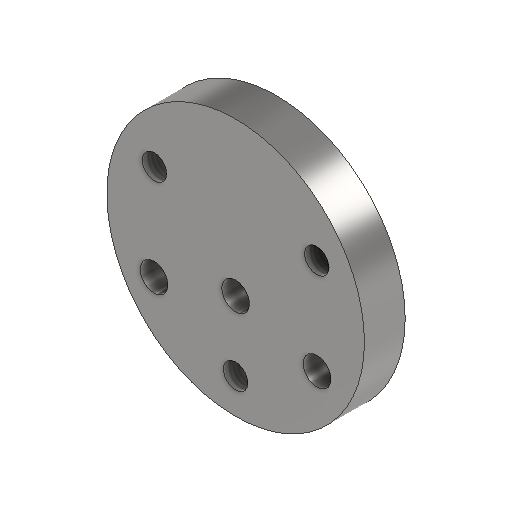
# Autodesk Inventor part: B_pipe_cylinder_5
Saved by Autodesk Inventor 2026.2 (Build 302298000, 298)
## iProperties
Created: 2026-02-02
Part Number: B_pipe_cylinder_5
Material: ステンレス鋼 440C
Document SubType Name: Modeling
Designer: zetsu
Density: 7.75 g/cm^3
Appearance: 半つや出し
Author: zetsu
Autodesk Inventor part; units mm, degrees
ref_plane "YZ Plane" through (0, 0, 0) normal (1, 0, 0) x (0, 1, 0)
ref_plane "XZ Plane" through (0, 0, 0) normal (0, 1, 0) x (-1, 0, 0)
ref_plane "XY Plane" through (0, 0, 0) normal (0, 0, 1) x (1, 0, 0)
sketch "スケッチ2" plane through (0, 0, 0) normal (0, 0, 1) x (1, 0, 0)
  circle A0 centre (0, 0) radius 15.8
  dimension "d0" = 31.6
  constraints: 1 centre point, 1 coincident
  measures "d0" diameter of A0
extrude "押し出し1" add sketch "スケッチ2" against normal blind 5
sketch "スケッチ3" plane through (0, 0, 0) normal (0, 0, 1) x (1, 0, 0)
  line L0 (0, 0) -> (0, 20.2537) construction
  circle A0 centre (0, -3) radius 1.7
  circle A1 centre (-10, -6) radius 1.7
  circle A2 centre (10, -6) radius 1.7
  dimension "d32" = 3.4
  dimension "d33" = 3
  dimension "d67" = 3.4
  dimension "d68" = 3.4
  dimension "d69" = 10
  dimension "d70" = 6
  constraints: 3 centre point, 2 end point, 1 symmetric about line, 1 vertical
  measures "d32" diameter of A0
  measures "d33" distance of A0.centre L0.start
  measures "d67" diameter of A1
  measures "d68" diameter of A2
  measures "d69" horizontal distance of L0.start A2.centre
  measures "d70" vertical distance of A2.centre L0.start
extrude "押し出し2" cut sketch "スケッチ3" against normal through all
sketch "スケッチ10" plane through (0, 0, 0) normal (0, 0, 1) x (1, 0, 0)
  circle A0 centre (0, -11.5) radius 1.5
  circle A1 centre (9.9593, 5.75) radius 1.5
  circle A2 centre (-9.9593, 5.75) radius 1.5
  point P0 (0, 0)
  dimension "d71" = 3
  dimension "d72" = 11.5
  dimension "d75" = 360
  constraints: 3 centre point, 7 other
  measures "d71" diameter of A0
  measures "d72" distance of A0.centre point (0, 0)
extrude "押し出し8" cut sketch "スケッチ10" against normal through all
thread "ねじ6" size "M3x0.5" class "6H" standard "ANSI Metric M Profile" full length
thread "ねじ7" size "M3x0.5" class "6H" standard "ANSI Metric M Profile" full length
thread "ねじ8" size "M3x0.5" class "6H" standard "ANSI Metric M Profile" full length
